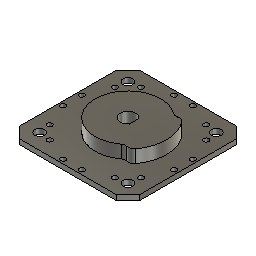
Nema 17 stepper motor encoder v4 (Autodesk Fusion 360 design; units mm, degrees)
Autodesk Fusion 360 part; units mm, degrees
note: some values were not read from the file. Set by a fixed rule: which sketch regions a step uses.
sketch "Sketch1" plane through (0, 0, 0) normal (0, 0, 1) x (1, 0, 0)
  line L0 (21, 21) -> (-21, 21)
  line L1 (-21, 21) -> (-21, -21)
  line L2 (-21, -21) -> (21, -21)
  line L3 (21, -21) -> (21, 21)
  line L4 (21, 21) -> (-21, -21) construction
  line L5 (-21, 21) -> (21, -21) construction
  circle A0 centre (0, 0) radius 11.25
  line L6 (0, 0) -> (0, 21) construction
  line L7 (0, 0) -> (21, 0) construction
  circle A1 centre (-15.5, 15.5) radius 1.75
  circle A2 centre (15.5, 15.5) radius 1.75
  circle A3 centre (-15.5, -15.5) radius 1.75
  circle A4 centre (15.5, -15.5) radius 1.75
  circle A5 centre (-3.25, 19.5) radius 0.9
  circle A6 centre (3.25, 19.5) radius 0.9
  circle A7 centre (-11.4905, 16.0867) radius 0.9
  circle A8 centre (-16.0867, 11.4905) radius 0.9
  circle A9 centre (-19.5, 3.25) radius 0.9
  circle A10 centre (-19.5, -3.25) radius 0.9
  circle A11 centre (-16.0867, -11.4905) radius 0.9
  circle A12 centre (-11.4905, -16.0867) radius 0.9
  circle A13 centre (-3.25, -19.5) radius 0.9
  circle A14 centre (3.25, -19.5) radius 0.9
  circle A15 centre (11.4905, -16.0867) radius 0.9
  circle A16 centre (16.0867, -11.4905) radius 0.9
  circle A17 centre (19.5, -3.25) radius 0.9
  circle A18 centre (19.5, 3.25) radius 0.9
  circle A19 centre (16.0867, 11.4905) radius 0.9
  circle A20 centre (11.4905, 16.0867) radius 0.9
  dimension "d2" = 42
  dimension "d3" = 42
  dimension "d5" = 22.5
  dimension "d8" = 31
  dimension "d9" = 3.5
  dimension "d10" = 1.8
  dimension "d12" = 6.5
  dimension "d17" = 360
  dimension "d41" = 19.5
  dimension "d42" = 1.5
  constraint horizontal L0
  constraint perpendicular L0 L1
  constraint parallel L0 L2
  constraint parallel L1 L3
  constraint coincident L4 A0.centre
  constraint coincident L5 A0.centre
  constraint coincident A0.centre L6.start
  constraint midpoint L0 L6.end
  constraint midpoint L3 L7.end
  constraint coincident L5 A1.centre
  constraint symmetric L6 A1 A2
  constraint symmetric L7 A1 A3
  constraint symmetric L7 A2 A4
  constraint symmetric L6 A5 A6
  measures "d2" distance of L1.end L2.end
  measures "d3" distance of L0.end L1.end
  measures "d5" diameter of A0
  measures "d8" distance of A1.centre A2.centre
  measures "d9" diameter of A1
  measures "d10" diameter of A5
  measures "d12" distance of A5.centre A6.centre
  measures "d41" vertical distance of A0.centre A6.centre
  measures "d42" distance of L0 A6.centre
extrude "Extrude1" add sketch "Sketch1" along normal blind 1.8 makes body 1
sketch "Sketch2" plane through (0, 0, 1.8) normal (0, 0, 1) x (-1, 0, 0)
  circle A0 centre (0, 0) radius 11.25 construction
  circle A1 centre (0, 0) radius 2.7
  line L0 (-6.4, -14.5) -> (6.4, -14.5) construction
  line L1 (6.4, -14.5) -> (6.4, -21) construction
  line L2 (-6.4, -21) -> (-6.4, -14.5) construction
  line L3 (-6.4, -14.5) -> (6.4, -21) construction
  line L4 (6.4, -14.5) -> (-6.4, -21) construction
  line L5 (6.4, -14.5) -> (-7.5453, -12.0411) construction
  circle A2 centre (0, 0) radius 11.5
  circle A3 centre (0, 0) radius 13.5
  circle A4 centre (-11.4905, 16.0867) radius 0.9
  circle A5 centre (11.4905, 16.0867) radius 0.9
  circle A6 centre (-16.0867, 11.4905) radius 0.9
  circle A7 centre (19.5, 3.25) radius 0.9
  circle A8 centre (-16.0867, -11.4905) radius 0.9
  circle A9 centre (-19.5, -3.25) radius 0.9
  circle A10 centre (-11.4905, -16.0867) radius 0.9
  circle A11 centre (-3.25, 19.5) radius 0.9
  circle A12 centre (3.25, 19.5) radius 0.9
  circle A13 centre (16.0867, 11.4905) radius 0.9
  circle A14 centre (-19.5, 3.25) radius 0.9
  circle A15 centre (19.5, -3.25) radius 0.9
  line L6 (-2, -1.8138) -> (-2, 1.8138) construction
  line L7 (14.7785, -5.7276) -> (19.3747, -10.3238) construction
  line L8 (5.7276, -14.7785) -> (14.7785, -5.7276) construction
  line L9 (10.3238, -19.3747) -> (5.7276, -14.7785) construction
  line L10 (14.7785, -5.7276) -> (3.179, -13.8497) construction
  line L11 (14.5, 6.4) -> (21, 6.4) construction
  line L12 (14.5, -6.4) -> (14.5, 6.4) construction
  line L13 (21, -6.4) -> (14.5, -6.4) construction
  line L14 (14.5, 6.4) -> (12.0411, -7.5453) construction
  line L15 (5.7276, 14.7785) -> (10.3238, 19.3747) construction
  line L16 (14.7785, 5.7276) -> (5.7276, 14.7785) construction
  line L17 (19.3747, 10.3238) -> (14.7785, 5.7276) construction
  line L18 (5.7276, 14.7785) -> (13.8497, 3.179) construction
  line L19 (-6.4, 14.5) -> (-6.4, 21) construction
  line L20 (6.4, 14.5) -> (-6.4, 14.5) construction
  line L21 (6.4, 21) -> (6.4, 14.5) construction
  line L22 (-6.4, 14.5) -> (7.5453, 12.0411) construction
  line L23 (-14.7785, 5.7276) -> (-19.3747, 10.3238) construction
  line L24 (-5.7276, 14.7785) -> (-14.7785, 5.7276) construction
  line L25 (-10.3238, 19.3747) -> (-5.7276, 14.7785) construction
  line L26 (-14.7785, 5.7276) -> (-3.179, 13.8497) construction
  line L27 (-14.5, -6.4) -> (-21, -6.4) construction
  line L28 (-14.5, 6.4) -> (-14.5, -6.4) construction
  line L29 (-21, 6.4) -> (-14.5, 6.4) construction
  line L30 (-14.5, -6.4) -> (-12.0411, 7.5453) construction
  line L31 (-5.7276, -14.7785) -> (-10.3238, -19.3747) construction
  line L32 (-14.7785, -5.7276) -> (-5.7276, -14.7785) construction
  line L33 (-19.3747, -10.3238) -> (-14.7785, -5.7276) construction
  line L34 (-5.7276, -14.7785) -> (-13.8497, -3.179) construction
  line L35 (-21, -21) -> (21, -21)
  circle A16 centre (0, 0) radius 2.5 construction
  line L36 (-2.2, -1.5652) -> (-2.2, 1.5652)
  line L37 (-9.5459, -9.5459) -> (9.5459, 9.5459)
  line L38 (0, 0) -> (-13.5, 0) construction
  line L39 (-9.5459, 9.5459) -> (9.5459, -9.5459)
  point P0 (0, -17.75)
  dimension "d19" = 6.5
  dimension "d20" = 12.8
  dimension "d21" = 10
  dimension "d23" = 27
  dimension "d39" = 360
  dimension "d43" = 2
  dimension "d44" = 5
  dimension "d45" = 0.2
  dimension "d46" = 4.5
  dimension "d47" = 0.2
  dimension "d48" = 90
  constraint concentric A0 A1
  constraint horizontal L0
  constraint perpendicular L0 L1
  constraint parallel L1 L2
  constraint coincident L3 P0
  constraint coincident L4 P0
  constraint vertical A0.centre P0
  constraint concentric A0 A2
  constraint concentric A1 A3
  constraint coincident A1 L6.start
  constraint coincident A1 L6.end
  constraint coincident L2.start L35
  constraint coincident L1.end L35
  constraint concentric A2 A16
  constraint coincident A1 L36.start
  constraint coincident A1 L36.end
  constraint parallel L6 L36
  constraint vertical L36
  constraint coincident A3 L37.start
  constraint coincident A3 L37.end
  constraint coincident A0.centre L37
  constraint coincident A0.centre A1.centre
  constraint coincident A3 L38.end
  constraint horizontal L38
  constraint symmetric L37.start L38 L39.start
  constraint symmetric L37.end L38 L39.end
  measures "d19" distance of L0.start L2.start
  measures "d20" distance of L0.start L0.end
  measures "d21" angle of L0 L5
  measures "d23" diameter of A3
  measures "d43" distance of A2 A3
  measures "d44" diameter of A16
  measures "d45" distance of A1 A16
  measures "d47" distance of L6 L36
  measures "d48" angle of L37 L39
extrude "Extrude2" add sketch "Sketch2" along normal blind 4.5 separate body contours A1 L36 | A1 A2 L37 L39 | A1 A2 L37 L39 | A1 A2 L37 L39 | A1 A2 L37 L39 | A2 A3 L37 L39 picked at (-9.495, -8.5893) makes body 2
sketch "Sketch3" plane through (0, 0, 0) normal (1, 0, 0) x (0, 1, 0)
  line L0 (0, 6.3) -> (0, 1.8) construction
  circle A0 centre (0, 4.05) radius 0.9
  circle A1 centre (0, 4.05) radius 1.95
  line L1 (11.5, 6.3) -> (-11.5, 6.3)
  line L2 (11.5, 1.8) -> (-11.5, 1.8)
  point P0 (0, 1.8)
  point P1 (1.5652, 6.3)
  point P2 (-1.5652, 6.3)
  dimension "d29" = 1.8
  dimension "d30" = 3.9
  constraint coincident P0 L0.end
  constraint midpoint L0 A0.centre
  constraint concentric A0 A1
  constraint vertical L0
  measures "d29" diameter of A0
  measures "d30" diameter of A1
fillet "Fillet1" radius 2 4 edges at (8.1317, -8.1317, 4.05) (9.5459, -9.5459, 4.05) (8.1317, 8.1317, 4.05) (9.5459, 9.5459, 4.05) on bodies 2
chamfer "Chamfer1" distance 4 angle 45 4 edges at (-21, -21, 0.9) (-21, 21, 0.9) (21, -21, 0.9) (21, 21, 0.9) on bodies 1
equation "d2 = d3"
equation "d47 = d45"
